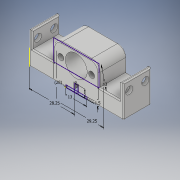
# Autodesk Inventor part: lead screw couple2
Saved by Autodesk Inventor 2018 (Build 220112000, 112)
## iProperties
Created: 2018-09-18
Part Number: lead screw couple2
Material: Generic
Document SubType Name: Modeling
Designer: Iek Man Lei
Density: 1 g/cm^3
Appearance: Default
Author: Iek Man Lei
Autodesk Inventor part; units mm, degrees
ref_plane "YZ Plane" through (0, 0, 0) normal (1, 0, 0) x (0, 1, 0)
ref_plane "XZ Plane" through (0, 0, 0) normal (0, 1, 0) x (-1, 0, 0)
ref_plane "XY Plane" through (0, 0, 0) normal (0, 0, 1) x (1, 0, 0)
sketch "Sketch1" plane through (0, 0, 0) normal (0, 1, 0) x (-1, 0, 0)
  line L0 (22.3889, 2.5556) -> (-36.1111, 2.5556)
  line L1 (-36.1111, 2.5556) -> (-36.1111, -14.4444)
  line L2 (-36.1111, -14.4444) -> (22.3889, -14.4444)
  line L3 (22.3889, -14.4444) -> (22.3889, 2.5556)
  point P0 (0, 0)
  dimension "d0" = 58.5
  dimension "d1" = 17
  constraints: 8 end point, 2 parallel, 1 horizontal, 1 perpendicular
  measures "d0" distance of L1.end L2.end
  measures "d1" distance of L0.end L1.end
extrude "Extrusion1" add sketch "Sketch1" along normal blind 10
sketch "Sketch2" plane through (36.1111, 0, -14.4444) normal (0, 0, -1) x (-1, 0, 0)
  point P0 (36.1111, 0)
sketch "Sketch3" plane through (0, 10, 0) normal (0, 1, 0) x (1, 0, 0)
  line L0 (36.1111, 14.4444) -> (-22.3889, 14.4444) projected
  line L1 (-22.3889, -2.5556) -> (36.1111, -2.5556) projected
  line L2 (-7.1389, 14.4444) -> (20.8611, 14.4444)
  line L3 (20.8611, 14.4444) -> (20.8611, -2.5556)
  line L4 (20.8611, -2.5556) -> (-7.1389, -2.5556)
  line L5 (-7.1389, -2.5556) -> (-7.1389, 14.4444)
  line L6 (36.1111, -2.5556) -> (36.1111, 14.4444) projected
  point P0 (0, 0)
  dimension "d4" = 28
  dimension "d5" = 15.25
  constraints: 8 end point, 2 parallel, 2 point on line, 1 horizontal, 1 perpendicular
  measures "d4" distance of L3.end L4.end
  measures "d5" distance between parallel lines of L6 L3
extrude "Extrusion2" add sketch "Sketch3" along normal blind 13 contours L3 L1 L5 L0
sketch "Sketch4" plane through (36.1111, 0, -14.4444) normal (0, 0, -1) x (-1, 0, 0)
  line L0 (58.5, 0) -> (58.5, 10) projected
  line L1 (49.2125, 8) -> (19.05, 8)
  line L2 (19.75, 21.5) -> (46.0375, 21.5)
  line L3 (15.25, 23) -> (43.25, 23) projected
  circle A0 centre (29.25, 14.75) radius 6.75
  circle A1 centre (38.75, 14.75) radius 1.85
  circle A2 centre (19.75, 14.75) radius 1.85
  circle A3 centre (29.25, 14.75) radius 7.5
  line L4 (40.0667, 21.5) -> (18.4333, 21.5)
  line L5 (18.4333, 21.5) -> (18.4333, 8)
  line L6 (18.4333, 8) -> (40.0667, 8)
  line L7 (40.0667, 8) -> (40.0667, 21.5)
  arc A4 (18.4333, 21.5) -> (18.4333, 8) centre (29.25, 14.75) ccw
  arc A5 (40.0667, 8) -> (40.0667, 21.5) centre (29.25, 14.75) ccw
  line L8 (0, 0) -> (0, 10) projected
  line L9 (58.5, 0) -> (0, 0) projected
  point P0 (36.1111, 0)
  dimension "d10" = 13.5
  dimension "d12" = 1.5
  dimension "d13" = 13.5
  dimension "d16" = 3.7
  dimension "d17" = 3.7
  dimension "d18" = 19
  dimension "d22" = 15
  dimension "d73" = 29.25
  dimension "d74" = 9.5
  dimension "d98" = 14.75
  constraints: 12 end point, 6 centre point, 4 point on circle, 3 coincident, 3 horizontal, 2 horizontal alignment, 2 parallel, 2 point on line, 1 perpendicular
  measures "d10" distance between parallel lines of L2 L1
  measures "d12" distance between parallel lines of L3 L2
  measures "d13" diameter of A0
  measures "d16" diameter of A1
  measures "d17" diameter of A2
  measures "d18" distance of A2.centre A1.centre
  measures "d22" diameter of A3
  measures "d73" distance from line of L8 A0.centre
  measures "d74" distance of A2.centre A0.centre
  measures "d98" distance from line of L9 A0.centre
extrude "Extrusion3" cut sketch "Sketch4" against normal through all contours L7 A1 | A1 L7 | A0 | L5 A2 | A2 L5
sketch "Sketch5" plane through (-22.3889, 0, 2.5556) normal (0, 0, 1) x (1, 0, 0)
  line L0 (43.25, 23) -> (15.25, 23) projected
  line L1 (43.25, 10) -> (43.25, 23) projected
  line L2 (15.25, 23) -> (43.25, 23)
  line L3 (43.25, 23) -> (43.25, 10)
  line L4 (43.25, 10) -> (15.25, 10)
  line L5 (15.25, 10) -> (15.25, 23)
  point P0 (22.3889, 0)
  dimension "d57" = 28
  constraints: 8 end point, 2 parallel, 1 horizontal, 1 perpendicular
  measures "d57" distance of L1.start L4.end
extrude "Extrusion6" cut sketch "Sketch4" against normal blind 6 from surface at 0 contours L1 A3 L2 L7 A1 | L7 A1 A5 | L1 A0 L2 A3 | L7 A1 | A1 L7 | L1 A3 L2 A0 | L1 L6 L5 A2 L4 L2 A3 | A4 L5 A2 | L5 A2 | A2 L5
fillet "Fillet1" radius 5 2 edges at (20.8611, 23, -5.9444) (-7.1389, 23, -5.9444)
sketch "Sketch6" plane through (36.1111, 0, -14.4444) normal (0, 0, -1) x (-1, 0, 0)
  circle A0 centre (29.25, 0) radius 6.5
  line L0 (58.5, 0) -> (58.5, 10) projected
  point P0 (36.1111, 0)
  dimension "d28" = 13
  dimension "d29" = 29.25
  constraints: 1 centre point
  measures "d28" diameter of A0
  measures "d29" distance from line of L0 A0.centre
extrude "Extrusion7" cut sketch "Sketch6" against normal blind 12
sketch "Sketch7" plane through (-22.3889, 0, 2.5556) normal (0, 0, 1) x (1, 0, 0)
  line L0 (22.75, 0) -> (35.75, 0) projected
  line L1 (30.25, 5) -> (28.25, 5)
  line L2 (28.25, 5) -> (28.25, 0)
  line L3 (28.25, 0) -> (30.25, 0)
  line L4 (30.25, 0) -> (30.25, 5)
  line L5 (0, 0) -> (0, 10) projected
  line L6 (22.75, 0) -> (35.75, 0)
  line L7 (35.75, 0) -> (35.75, 1.5)
  line L8 (35.75, 1.5) -> (22.75, 1.5)
  line L9 (22.75, 1.5) -> (22.75, 0)
  point P0 (22.3889, 0)
  point P1 (29.25, 0)
  dimension "d35" = 5
  dimension "d36" = 2
  dimension "d37" = 28.25
  dimension "d38" = 1.5
  dimension "d99" = 13
  constraints: 16 end point, 4 parallel, 2 horizontal, 2 perpendicular, 1 horizontal alignment, 1 midpoint
  measures "d35" distance of L3.end L1.start
  measures "d36" distance of L1.start L1.end
  measures "d37" distance between parallel lines of L5 L2
  measures "d38" distance of L6.end L7.end
  measures "d99" distance between parallel lines of L9 L7
extrude "Extrusion8" cut sketch "Sketch7" against normal blind 11
extrude "Extrusion9" add sketch "Sketch6" against normal blind 10
sketch "Sketch8" plane through (-22.3889, 0, -14.4444) normal (0, 0, -1) x (-1, 0, 0)
  line L0 (0, 0) -> (-58.5, 0) projected
  line L1 (-16, -7.9375) -> (-42.8625, -7.9375)
  line L2 (-42.8625, -7.9375) -> (-42.8625, 0)
  line L3 (-42.8625, 0) -> (-16, 0)
  line L4 (-16, 0) -> (-16, -7.9375)
  line L5 (0, 0) -> (0, 10) projected
  point P0 (-22.3889, 0)
  point P1 (-35.75, 0)
  dimension "d75" = 16
  constraints: 8 end point, 2 parallel, 1 horizontal, 1 perpendicular, 1 point on line
  measures "d75" distance between parallel lines of L5 L4
extrude "Extrusion10" cut sketch "Sketch8" against normal through all
sketch "Sketch10" plane through (36.1111, 0, -14.4444) normal (0, 0, -1) x (-1, 0, 0)
  point P0 (36.1111, 0)
sketch "Sketch12" plane through (0, 0, 0) normal (0, -1, 0) x (1, 0, 0)
  line L0 (-4.4889, -8.4444) -> (-4.4889, 2.5556) projected
  circle A0 centre (-4.1389, -0.9444) radius 2.25
  circle A1 centre (-13.1389, -10.9444) radius 2.25
  circle A2 centre (17.8611, -0.9444) radius 2.25
  circle A3 centre (26.8611, -10.9444) radius 2.25
  line L1 (-22.3889, 2.5556) -> (36.1111, 2.5556) projected
  line L2 (36.1111, -14.4444) -> (-22.3889, -14.4444) projected
  line L3 (36.1111, 2.5556) -> (36.1111, -14.4444) projected
  point P0 (0, 0)
  point P1 (13.3611, 2.5556)
  point P2 (15.6111, 2.5556)
  dimension "d58" = 4.5
  dimension "d59" = 4.5
  dimension "d60" = 4.5
  dimension "d61" = 4.5
  dimension "d62" = 3.5
  dimension "d63" = 3.5
  dimension "d64" = 22
  dimension "d65" = 40
  dimension "d76" = 9.25
  dimension "d77" = 9
  constraints: 4 centre point, 2 horizontal alignment
  measures "d58" diameter of A0
  measures "d59" diameter of A1
  measures "d60" diameter of A2
  measures "d61" diameter of A3
  measures "d62" distance from line of L1 A2.centre
  measures "d63" distance from line of L2 A3.centre
  measures "d64" distance of A0.centre A2.centre
  measures "d65" distance of A1.centre A3.centre
  measures "d76" distance from line of L3 A3.centre
  measures "d77" horizontal distance of A3.centre A2.centre
extrude "Extrusion13" cut sketch "Sketch12" against normal blind 3.5
fillet "Fillet3" radius 0.5 5 edges at (6.8611, 23, -14.4444) (-5.6744, 21.5355, -14.4444) (-7.1389, 14, -14.4444) (20.8611, 14, -14.4444) (19.3966, 21.5355, -14.4444)
fillet "Fillet4" radius 0.5 10 edges at (5.8611, 1.5, 0.0556) (7.8611, 1.5, 0.0556) (3.1988, 1.5, -2.4444) (10.5234, 1.5, -2.4444) (5.8611, 3.25, 2.5556) (6.8611, 5, 2.5556) (7.8611, 3.25, 2.5556) (5.8611, 3.25, -2.4444) (6.8611, 5, -2.4444) (7.8611, 3.25, -2.4444)
sketch "Sketch13" plane through (0, 0, 0) normal (0, -1, 0) x (1, 0, 0)
  point P0 (0, 0)
sketch "Sketch14" plane through (0, 10, 0) normal (0, 1, 0) x (1, 0, 0)
  line L0 (-22.3889, -2.5556) -> (-7.1389, -2.5556) projected
  line L1 (36.1111, 14.4444) -> (-22.3889, 14.4444) projected
  line L2 (-22.3889, -2.5556) -> (-20.3889, -2.5556)
  line L3 (-20.3889, -2.5556) -> (-20.3889, 14.4444)
  line L4 (-20.3889, 14.4444) -> (-22.3889, 14.4444)
  line L5 (-22.3889, 14.4444) -> (-22.3889, -2.5556)
  line L6 (13.3611, -2.5556) -> (36.1111, -2.5556) projected
  line L7 (36.1111, 14.4444) -> (34.1111, 14.4444)
  line L8 (34.1111, 14.4444) -> (34.1111, -2.5556)
  line L9 (34.1111, -2.5556) -> (36.1111, -2.5556)
  line L10 (36.1111, -2.5556) -> (36.1111, 14.4444)
  point P0 (0, 0)
  dimension "d78" = 2
  dimension "d79" = 2
  constraints: 16 end point, 4 parallel, 2 horizontal, 2 perpendicular, 2 point on line
  measures "d78" distance of L4.end L3.end
  measures "d79" distance of L9.end L8.end
extrude "Extrusion14" add sketch "Sketch14" along normal blind 10
sketch "Sketch15" plane through (36.1111, 0, 2.5556) normal (1, 0, 0) x (0, 0, -1)
  circle A0 centre (3.5, 14.5) radius 2.25
  circle A1 centre (13.5, 14.5) radius 2.25
  line L0 (0, 10) -> (17, 10) projected
  line L1 (17, 0) -> (17, 20) projected
  point P0 (2.5556, 0)
  dimension "d82" = 4.5
  dimension "d83" = 4.5
  dimension "d84" = 10
  dimension "d85" = 4.5
  dimension "d86" = 3.5
  constraints: 2 centre point, 1 horizontal alignment
  measures "d82" diameter of A0
  measures "d83" diameter of A1
  measures "d84" distance of A0.centre A1.centre
  measures "d85" distance from line of L0 A0.centre
  measures "d86" distance from line of L1 A1.centre
extrude "Extrusion15" cut sketch "Sketch15" against normal blind 3
sketch "Sketch16" plane through (-22.3889, 0, -14.4444) normal (-1, 0, 0) x (0, 0, 1)
  circle A0 centre (3.5, 14.5) radius 2.25
  circle A1 centre (13.5, 14.5) radius 2.25
  line L0 (0, 0) -> (0, 20) projected
  line L1 (0, 10) -> (17, 10) projected
  point P0 (14.4444, 0)
  dimension "d89" = 4.5
  dimension "d90" = 4.5
  dimension "d91" = 10
  dimension "d92" = 3.5
  dimension "d93" = 4.5
  constraints: 2 centre point, 1 horizontal alignment
  measures "d89" diameter of A0
  measures "d90" diameter of A1
  measures "d91" distance of A0.centre A1.centre
  measures "d92" distance from line of L0 A0.centre
  measures "d93" distance from line of L1 A1.centre
extrude "Extrusion16" cut sketch "Sketch16" against normal blind 3
fillet "Fillet5" radius 0.7 26 edges at (-13.5139, 10, -14.4444) (-20.3889, 15, -14.4444) (-20.3889, 20, -5.9444) (-22.3889, 20, -5.9444) (-22.3889, 10, -14.4444) (-11.0139, 0, -14.4444) (24.7361, 0, -14.4444) (6.8611, 0, -14.4444) (36.1111, 10, -14.4444) (36.1111, 20, -5.9444) (36.1111, 10, 2.5556) (36.1111, 0, -5.9444) (34.1111, 20, -5.9444) (27.4861, 10, 2.5556) (27.2361, 10, -14.4444) (34.1111, 15, -14.4444) (24.7361, 0, 2.5556) (-11.0139, 0, 2.5556) (-22.3889, 10, 2.5556) (-13.7639, 10, 2.5556) (-20.3889, 15, 2.5556) (6.8611, 23, 2.5556) (19.3966, 21.5355, 2.5556) (20.8611, 14, 2.5556) (-7.1389, 14, 2.5556) (-5.6744, 21.5355, 2.5556)
fillet "Fillet6" radius 0.7 3 edges at (-22.1839, 0.205, 2.3505) (-22.1839, 0.205, -14.2394) (-22.3889, 0, -5.9444)
body "Solid1"
